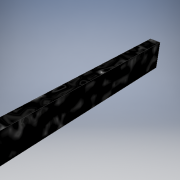
# Autodesk Inventor part: PinHeader-Female(LowPoly)
Saved by Autodesk Inventor 2018 (Build 220112000, 112)
## iProperties
Created: 2025-02-19
Part Number: PinHeader-Female(LowPoly)
Material: Všeobecné
Document SubType Name: Modeling
Designer: Jozko Mrkvicka
Density: 1 g/cm^3
Appearance: Výchozí
Author: Jozko Mrkvicka
Autodesk Inventor part; units mm, degrees
ref_plane "YZ Plane" through (0, 0, 0) normal (1, 0, 0) x (0, 1, 0)
ref_plane "XZ Plane" through (0, 0, 0) normal (0, 1, 0) x (-1, 0, 0)
ref_plane "XY Plane" through (0, 0, 0) normal (0, 0, 1) x (1, 0, 0)
sketch "Náčrt1" plane through (0, 0, 0) normal (0, 1, 0) x (-1, 0, 0)
  line L0 (-40.64, 2.54) -> (40.64, 2.54)
  line L1 (40.64, 2.54) -> (40.64, -2.54)
  line L2 (40.64, -2.54) -> (-40.64, -2.54)
  line L3 (-40.64, -2.54) -> (-40.64, 2.54)
  line L4 (-40.64, 2.54) -> (40.64, -2.54) construction
  line L5 (40.64, 2.54) -> (-40.64, -2.54) construction
  point P0 (0, 0)
  dimension "d0" = 81.28
  dimension "d1" = 5.08
  constraints: 12 end point, 2 midpoint, 2 parallel, 1 horizontal, 1 perpendicular
  measures "d0" distance of L1.end L2.end
  measures "d1" distance of L0.end L1.end
extrude "Vysunutí1" add sketch "Náčrt1" along normal blind 12.7
equation "\"d2\" = gPinHeaderHeight + gPcbThickness"
equation "\"thickness\" = 2.54"
equation "\"gPinHeaderHeight\" = 10.16"
equation "\"gPcbThickness\" = 2.54"
